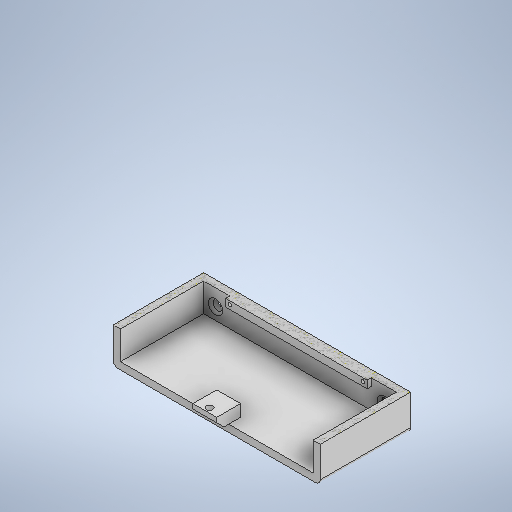
# Autodesk Inventor part: Backboard deel 1
Saved by Autodesk Inventor 2025.2 (Build 292293000, 293)
## iProperties
Created: 2024-12-12
Part Number: Backboard deel 1
Material: Generic
Document SubType Name: Modeling
Designer: jurre
Density: 1 g/cm^3
Appearance: Default
Author: jurre
Autodesk Inventor part; units mm, degrees
ref_plane "YZ Plane" through (0, 0, 0) normal (1, 0, 0) x (0, 1, 0)
ref_plane "XZ Plane" through (0, 0, 0) normal (0, 1, 0) x (-1, 0, 0)
ref_plane "XY Plane" through (0, 0, 0) normal (0, 0, 1) x (1, 0, 0)
sketch "Sketch1" plane through (0, 0, 0) normal (0, 0, 1) x (1, 0, 0)
  line L0 (25.0097, 21.6893) -> (25.0097, -75.3107)
  line L1 (-44.9903, 13.4393) -> (14.5097, 13.4393)
  line L2 (14.5097, 13.4393) -> (14.5097, -66.5607)
  line L3 (14.5097, -66.5607) -> (-44.9903, -66.5607)
  line L4 (-44.9903, -66.5607) -> (-44.9903, 13.4393)
  circle A0 centre (12.7597, 11.6893) radius 0.75
  circle A1 centre (-43.2403, 11.6893) radius 0.75
  circle A2 centre (-43.2403, -64.8107) radius 0.75
  circle A3 centre (12.7597, -64.8107) radius 0.75
  line L5 (-44.9903, 13.4393) -> (14.5097, 13.4393)
  line L6 (14.5097, 13.4393) -> (14.5097, 9.9393)
  line L7 (14.5097, 9.9393) -> (-44.9903, 9.9393)
  line L8 (-44.9903, 9.9393) -> (-44.9903, 13.4393)
  line L9 (14.5097, -66.5607) -> (-44.9903, -66.5607)
  line L10 (-44.9903, -66.5607) -> (-44.9903, -63.0607)
  line L11 (-44.9903, -63.0607) -> (14.5097, -63.0607)
  line L12 (14.5097, -63.0607) -> (14.5097, -66.5607)
  circle A4 centre (-50.9903, 20.1893) radius 2
  circle A5 centre (20.0097, 20.1893) radius 2
  circle A6 centre (20.0097, -70.3107) radius 2
  circle A7 centre (-50.9903, -70.3107) radius 2
  line L13 (-55.9903, 25.6893) -> (25.0097, 25.6893)
  line L14 (25.0097, 25.6893) -> (25.0097, -75.3107)
  line L15 (25.0097, -75.3107) -> (-55.9903, -75.3107)
  line L16 (-55.9903, -75.3107) -> (-55.9903, 25.6893)
  line L17 (-55.9903, 10.6893) -> (-55.9903, 17.6893)
  line L18 (25.0097, 10.1893) -> (25.0097, 17.1893)
  line L19 (-58.9903, 28.6893) -> (28.0097, 28.6893)
  line L20 (28.0097, 28.6893) -> (28.0097, -78.3107)
  line L21 (28.0097, -78.3107) -> (-58.9903, -78.3107)
  line L22 (-58.9903, -78.3107) -> (-58.9903, 28.6893)
  point P0 (0, 0)
  point P1 (-14.9903, -76.5607)
  point P2 (-44.9903, 9.9393)
  point P3 (14.5097, 9.9393)
  point P4 (14.5097, -63.0607)
  point P5 (-44.9903, -63.0607)
  dimension "d4" = 10
  dimension "d5" = 10.5
  dimension "d6" = 1.5
  dimension "d7" = 1.5
  dimension "d8" = 1.5
  dimension "d9" = 1.5
  dimension "d11" = 1.75
  dimension "d12" = 1.75
  dimension "d13" = 1.75
  dimension "d14" = 1.75
  dimension "d15" = 1.75
  dimension "d16" = 1.75
  dimension "d17" = 1.75
  dimension "d18" = 1.75
  dimension "d20" = 0
  dimension "d21" = 0
  dimension "d22" = 3.5
  dimension "d24" = 0
  dimension "d25" = 3.5
  dimension "d26" = 0
  dimension "d39" = 4
  dimension "d42" = 4
  dimension "d43" = 4
  dimension "d44" = 4
  dimension "d46" = 5
  dimension "d47" = 5
  dimension "d70" = 81
  dimension "d71" = 101
  dimension "d75" = 5.5
  dimension "d111" = 87
  dimension "d112" = 107
  dimension "d113" = 3
  dimension "d114" = 3
  dimension "d115" = 5
  dimension "d116" = 5
  dimension "d117" = 5
  dimension "d125" = 3
  dimension "d126" = 5
  dimension "d127" = 5.5
  dimension "d128" = 11
  dimension "d129" = 3
  constraints: 46 end point, 10 parallel, 8 centre point, 5 horizontal, 5 perpendicular, 2 point on line
  measures "d4" distance from line of point (-14.99, -76.561) L3
  measures "d5" distance between parallel lines of L0 L2
  measures "d6" diameter of A0
  measures "d7" diameter of A1
  measures "d8" diameter of A2
  measures "d9" diameter of A3
  measures "d11" distance from line of L1 A1.centre
  measures "d12" distance from line of L4 A1.centre
  measures "d13" distance from line of L1 A0.centre
  measures "d14" distance from line of L2 A0.centre
  measures "d15" distance from line of L2 A3.centre
  measures "d16" distance from line of L3 A3.centre
  measures "d17" distance from line of L4 A2.centre
  measures "d18" distance from line of L3 A2.centre
  measures "d20" distance between parallel lines of L2 L6
  measures "d21" distance between parallel lines of L1 L5
  measures "d22" distance of L7.end L5.start
  measures "d24" distance between parallel lines of L2 L12
  measures "d25" distance of L11.end L9.start
  measures "d26" distance between parallel lines of L3 L9
  measures "d39" diameter of A4
  measures "d42" diameter of A5
  measures "d43" diameter of A6
  measures "d44" diameter of A7
  measures "d46" distance from line of L0 A5.centre
  measures "d47" distance from line of L0 A6.centre
  measures "d70" distance of L13.start L13.end
  measures "d71" distance of L13.end L0.end
  measures "d75" distance from line of L13 A5.centre
  measures "d111" distance of L19.start L19.end
  measures "d112" distance of L19.end L20.end
  measures "d113" distance between parallel lines of L13 L19
  measures "d114" distance between parallel lines of L0 L20
  measures "d115" distance from line of L16 A7.centre
  measures "d116" distance from line of L15 A6.centre
  measures "d117" distance from line of L15 A7.centre
  measures "d125" distance between parallel lines of L22 L16
  measures "d126" distance from line of L16 A4.centre
  measures "d127" distance from line of L13 A4.centre
  measures "d128" distance between parallel lines of L16 L4
  measures "d129" distance between parallel lines of L21 L15
extrude "Extrusion5" add sketch "Sketch1" against normal blind 3 contours L0 L15 L16 L13 L14 | L1 L2 L7 L4 | L7 L2 L11 L4 | L11 L2 L3 L4 | A0 | A1 | A2 | A3 | A4 | A5 | A6 | A7 | L19 L20 L21 L22
extrude "Extrusion7" add sketch "Sketch1" along normal blind 1.75 contours L1 L2 L7 L4 | L11 L2 L3 L4
extrude "Extrusion11" cut sketch "Sketch1" against normal blind 200 contours A4 | A5 | A6 | A7
fillet "Fillet3" radius 1 4 edges at (-52.9903, 20.1893, 0) (18.0097, 20.1893, 0) (18.0097, -70.3107, 0) (-52.9903, -70.3107, 0)
extrude "Extrusion17" add sketch "Sketch1" along normal blind 35 contours L19 L20 L21 L22
sketch "Sketch9" plane through (-55.9903, -75.3107, 0) normal (1, 0, 0) x (0, 0, -1)
  line L0 (-35, 0) -> (-35, 101) projected
  line L1 (-35, 101) -> (-30.5, 101)
  line L2 (-30.5, 101) -> (-30.5, 89)
  line L3 (-30.5, 89) -> (-35, 89)
  line L4 (-35, 89) -> (-35, 101)
  point P0 (0, 75.3107)
  point P1 (-35, 89)
  dimension "d120" = 4.5
  dimension "d121" = 12
  constraints: 8 end point, 2 parallel, 1 horizontal, 1 perpendicular
  measures "d120" distance of L2.end L3.end
  measures "d121" distance of L1.end L2.end
extrude "Extrusion18" add sketch "Sketch9" along normal blind 81
fillet "Fillet4" radius 2 4 edges at (-58.9903, 28.6893, 16) (28.0097, 28.6893, 16) (28.0097, -78.3107, 16) (-58.9903, -78.3107, 16)
sketch "Sketch11" plane through (-55.9903, 13.6893, 30.5) normal (0, 0, -1) x (-1, 0, 0)
  line L0 (-71, 9) -> (-61, 9)
  line L1 (-61, 9) -> (-61, 3)
  line L2 (-61, 3) -> (-71, 3)
  line L3 (-71, 3) -> (-71, 9)
  line L4 (-81, 0) -> (-81, 12) projected
  line L5 (-81, 12) -> (0, 12) projected
  line L6 (0, 12) -> (0, 0) projected
  line L7 (-20, 9) -> (-10, 9)
  line L8 (-10, 9) -> (-10, 3)
  line L9 (-10, 3) -> (-20, 3)
  line L10 (-20, 3) -> (-20, 9)
  point P0 (-55.9903, -13.6893)
  dimension "d130" = 6
  dimension "d131" = 10
  dimension "d132" = 10
  dimension "d133" = 3
  dimension "d137" = 10
  dimension "d138" = 10
  dimension "d139" = 6
  dimension "d140" = 3
  constraints: 16 end point, 4 parallel, 2 horizontal, 2 perpendicular
  measures "d130" distance of L0.end L1.end
  measures "d131" distance between parallel lines of L4 L3
  measures "d132" distance of L0.start L0.end
  measures "d133" distance between parallel lines of L5 L0
  measures "d137" distance between parallel lines of L6 L8
  measures "d138" distance of L7.start L7.end
  measures "d139" distance of L9.end L7.start
  measures "d140" distance between parallel lines of L5 L7
extrude "Extrusion19" cut sketch "Sketch11" against normal blind 5
sketch "Sketch12" plane through (-55.9903, -75.3107, 0) normal (0, 1, 0) x (1, 0, 0)
  line L0 (35.5, -35) -> (45.5, -35)
  line L1 (45.5, -35) -> (45.5, -30)
  line L2 (45.5, -30) -> (35.5, -30)
  line L3 (35.5, -30) -> (35.5, -35)
  line L4 (0, 0) -> (0, -35) projected
  line L5 (81, -35) -> (0, -35) projected
  line L6 (81, 0) -> (81, -35) projected
  point P0 (55.9903, 0)
  dimension "d143" = 35.5
  dimension "d144" = 0
  dimension "d146" = 5
  dimension "d147" = 10
  dimension "d148" = 35.5
  constraints: 8 end point, 2 parallel, 1 horizontal, 1 perpendicular
  measures "d143" distance between parallel lines of L4 L3
  measures "d144" distance between parallel lines of L5 L0
  measures "d146" distance of L0.end L1.end
  measures "d147" distance of L1.end L2.end
  measures "d148" distance between parallel lines of L6 L1
extrude "Extrusion20" add sketch "Sketch12" along normal blind 5
sketch "Sketch13" plane through (0, 0, 35) normal (0, 0, 1) x (1, 0, 0)
  line L0 (-20.4903, -70.3107) -> (-10.4903, -70.3107) projected
  line L1 (-20.4903, -75.3107) -> (-10.4903, -75.3107) projected
  line L2 (-20.4903, -70.3107) -> (-10.4903, -70.3107)
  line L3 (-10.4903, -70.3107) -> (-10.4903, -75.3107)
  line L4 (-10.4903, -75.3107) -> (-20.4903, -75.3107)
  line L5 (-20.4903, -75.3107) -> (-20.4903, -70.3107)
  point P0 (0, 0)
  constraints: 8 end point, 2 parallel, 1 horizontal, 1 perpendicular
extrude "Extrusion21" add sketch "Sketch13" along normal blind 5
chamfer "Chamfer3" distance 3 angle 45 1 edges at (-15.4903, -75.3107, 40)
sketch "Sketch14" plane through (-55.9903, -70.3107, 0) normal (0, 1, 0) x (1, 0, 0)
  circle A0 centre (40.5, -38) radius 1.375
  line L0 (45.5, -30) -> (45.5, -40) projected
  line L1 (35.5, -30) -> (35.5, -40) projected
  line L2 (45.5, -30) -> (35.5, -30) projected
  line L3 (45.5, -40) -> (35.5, -40) projected
  point P0 (55.9903, 0)
  point P1 (40.5, -30)
  point P2 (40.5, -40)
  dimension "d156" = 2.75
  dimension "d157" = 5
  dimension "d158" = 5
  dimension "d159" = 8
  dimension "d160" = 2
  constraints: 2 midpoint, 1 centre point
  measures "d156" diameter of A0
  measures "d157" distance from line of L0 A0.centre
  measures "d158" distance from line of L1 A0.centre
  measures "d159" distance of point (40.5, -30) A0.centre
  measures "d160" distance of point (40.5, -40) A0.centre
extrude "Extrusion22" cut sketch "Sketch14" against normal blind 5 contours A0
body "Solid2"
